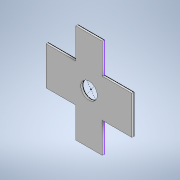
# Autodesk Inventor part: kill swich
Saved by Autodesk Inventor 2022 (Build 260153000, 153)
## iProperties
Created: 2022-03-09
Part Number: kill swich
Material: Genérico
Document SubType Name: Modeling
Designer: Guilherme
Density: 1 g/cm^3
Appearance: Padrão
Author: Guilherme
Autodesk Inventor part; units mm, degrees
ref_plane "YZ Plane" through (0, 0, 0) normal (1, 0, 0) x (0, 1, 0)
ref_plane "XZ Plane" through (0, 0, 0) normal (0, 1, 0) x (-1, 0, 0)
ref_plane "XY Plane" through (0, 0, 0) normal (0, 0, 1) x (1, 0, 0)
sketch "Esboço2" plane through (0, 0, 0) normal (0, 0, 1) x (1, 0, 0)
  line L0 (-20, 29) -> (20, 29)
  line L1 (20, 29) -> (20, -29)
  line L2 (20, -29) -> (-20, -29)
  line L3 (-20, -29) -> (-20, 29)
  line L4 (-20, 29) -> (20, -29) construction
  line L5 (20, 29) -> (-20, -29) construction
  line L6 (20, 29) -> (65, 29)
  line L7 (65, 29) -> (65, -29)
  line L8 (65, -29) -> (20, -29)
  line L9 (20, -29) -> (20, 29)
  line L10 (-20, 29) -> (-65, 29)
  line L11 (-65, 29) -> (-65, -29)
  line L12 (-65, -29) -> (-20, -29)
  line L13 (-20, -29) -> (-20, 29)
  circle A0 centre (0, 0) radius 12.5
  line L14 (-20, 29) -> (20, 29)
  line L15 (20, 29) -> (20, 75)
  line L16 (20, 75) -> (-20, 75)
  line L17 (-20, 75) -> (-20, 29)
  line L18 (-20, -29) -> (20, -29)
  line L19 (20, -29) -> (20, -75)
  line L20 (20, -75) -> (-20, -75)
  line L21 (-20, -75) -> (-20, -29)
  point P0 (20, -29)
  point P1 (20, 29)
  dimension "d1" = 40
  dimension "d2" = 58
  dimension "d3" = 45
  dimension "d4" = 45
  dimension "d5" = 25
  dimension "d6" = 46
  dimension "d7" = 46
  constraints: 44 end point, 10 parallel, 5 horizontal, 5 perpendicular, 2 midpoint, 1 centre point, 1 coincident, 1 point on line
  measures "d1" distance of L1.end L2.end
  measures "d2" distance of L0.end L1.end
  measures "d3" distance of L7.end L8.end
  measures "d4" distance of L12.end L11.end
  measures "d5" diameter of A0
  measures "d6" distance of L15.end L14.end
  measures "d7" distance of L18.end L19.end
extrude "Extrusão1" add sketch "Esboço2" along normal blind 3
